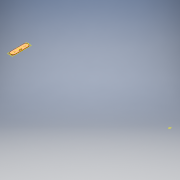
# Autodesk Inventor part: board
Saved by Autodesk Inventor 2017 SP1 (Build 210196100, 196)
## iProperties
Part Number: board
Material: 木材(サクラ)
Document SubType Name: Modeling
Designer: gisen
Density: 0.63 g/cm^3
Appearance: サクラ材 - ナチュラル 抑えた光沢
Mass: 1995.16 g
Surface Area: 3562.51 cm^2
Volume: 3166.92 cm^3
Author: gisen
Autodesk Inventor part; units mm, degrees
ref_plane "作業平面1" through (6614.749, 337.2794, 0) normal (0, 0, 1) x (1, 0, 0)
sketch "スケッチ1" plane through (6614.749, 337.2794, 0) normal (0, 0, 1) x (1, 0, 0)
  line L0 (-6509.749, -42.2794) -> (-6509.749, -632.2794)
  line L1 (-6509.749, -632.2794) -> (-6719.749, -632.2794)
  line L2 (-6719.749, -632.2794) -> (-6719.749, -42.2794)
  line L3 (-6719.749, -42.2794) -> (-6509.749, -42.2794)
  arc A0 (-6509.749, -42.2794) -> (-6719.749, -42.2794) centre (-6614.749, -42.2794) ccw
  arc A1 (-6719.749, -632.2794) -> (-6509.749, -632.2794) centre (-6614.749, -632.2794) ccw
  line L4 (-6614.749, -897.2794) -> (-6614.749, 222.7206) projected
  line L5 (-8036.2537, -337.2794) -> (1179.2797, -337.2794) projected
  line L6 (-6509.749, -337.2794) -> (-137.2251, -337.2794)
  point P0 (-6614.749, -337.2794)
  dimension "d1" = 210
  dimension "d3" = 105
  dimension "d4" = 590
  dimension "d5" = 105
  dimension "d8" = 295
  constraints: 10 end point, 4 point on circle, 2 centre point, 2 parallel, 2 perpendicular, 2 tangent, 1 collinear, 1 midpoint, 1 vertical
  measures "d1" distance of L0.end L1.end
  measures "d3" radius of A0
  measures "d4" distance between parallel lines of L1 L3
  measures "d5" distance between parallel lines of L0 L4
  measures "d8" distance between parallel lines of L6 L1
extrude "押し出し1" add sketch "スケッチ1" along normal blind 20
sketch "スケッチ2" plane through (6614.749, 337.2794, 0) normal (0, 0, -1) x (-1, 0, 0)
  spline S0 degree 3 poles (6630.8363, -557.2765) (6630.8356, -556.4314) (6630.8307, -555.5861) (6630.7821, -551.1548) (6630.6652, -547.5706) (6630.2129, -540.6292) (6629.8924, -537.269) (6629.059, -531.5504) (6628.6277, -529.1809) (6627.5, -524.5004) (6626.8057, -522.1844) (6625.8839, -519.9595) knots -3.785676 -3.785676 -3.785676 -3.785676 -3.532131 -3.532131 -2.4562 -2.4562 -1.444966 -1.444966 -0.722485 -0.722485 0 0 0 0
  spline S1 degree 3 poles (6630.0302, -579.9499) (6630.1435, -578.1819) (6630.247, -576.4134) (6630.4408, -572.7081) (6630.5289, -570.7713) (6630.6019, -568.834) (6630.6759, -566.8669) (6630.7344, -564.8993) (6630.8129, -561.0466) (6630.8346, -559.1616) (6630.8363, -557.2765) knots -2.294162 -2.294162 -2.294162 -2.294162 -1.762693 -1.762693 -1.181069 -1.181069 -1.181069 -0.590534 -0.590534 -0.025021 -0.025021 -0.025021 -0.025021
  spline S2 degree 3 poles (6629.9005, -581.946) (6629.933, -581.4474) (6629.9654, -580.9489) (6629.9979, -580.4504) (6630.0033, -580.367) (6630.0087, -580.2836) (6630.0195, -580.1167) (6630.0249, -580.0333) (6630.0302, -579.9499) knots 0 0 0 0 0.749256 0.749256 0.749256 0.874628 0.874628 1 1 1 1
  ellipse E0 centre (6627.749, -583.7463) end of major axis (6627.749, -580.2108) minor radius 2.5 (6630.249, -583.7463) -> (6629.9005, -581.946) ccw
  line L0 (6630.249, -596.9595) -> (6630.249, -583.7463)
  line L1 (6640.249, -596.9595) -> (6630.249, -596.9595)
  arc A0 (6640.249, -596.9595) -> (6641.749, -595.4595) centre (6640.249, -595.4595) ccw
  line L2 (6641.749, -521.4595) -> (6641.749, -595.4595)
  arc A1 (6641.749, -521.4595) -> (6640.249, -519.9595) centre (6640.249, -521.4595) ccw
  line L3 (6625.8839, -519.9595) -> (6640.249, -519.9595)
  circle A2 centre (6635.249, -591.4595) radius 3
  circle A3 centre (6635.249, -528.4595) radius 3
  circle A4 centre (6594.249, -591.4595) radius 3
  circle A5 centre (6594.249, -528.4595) radius 3
  spline S3 degree 3 poles (6599.4677, -579.9499) (6599.473, -580.0333) (6599.4784, -580.1167) (6599.4892, -580.2836) (6599.4946, -580.367) (6599.5, -580.4504) (6599.5325, -580.9489) (6599.5649, -581.4474) (6599.5974, -581.946) knots 0 0 0 0 0.125372 0.125372 0.250745 0.250745 0.250745 1 1 1 1
  spline S4 degree 3 poles (6598.6616, -557.2765) (6598.6633, -559.1539) (6598.6848, -561.0313) (6598.7628, -564.8687) (6598.8208, -566.8287) (6598.8943, -568.7881) (6598.9673, -570.7332) (6599.0556, -572.6776) (6599.25, -576.3981) (6599.3539, -578.1743) (6599.4677, -579.9499) knots -2.319296 -2.319296 -2.319296 -2.319296 -1.756075 -1.756075 -1.167834 -1.167834 -1.167834 -0.583917 -0.583917 -0.050156 -0.050156 -0.050156 -0.050156
  spline S5 degree 3 poles (6603.614, -519.9595) (6602.3019, -523.1265) (6601.4408, -526.4662) (6600.1974, -532.85) (6599.7845, -535.9073) (6599.0649, -543.0901) (6598.8445, -547.2235) (6598.6873, -553.3316) (6598.6634, -555.3041) (6598.6616, -557.2765) knots -3.810629 -3.810629 -3.810629 -3.810629 -2.782212 -2.782212 -1.858006 -1.858006 -0.616716 -0.616716 -0.024978 -0.024978 -0.024978 -0.024978
  line L4 (6589.249, -519.9595) -> (6603.614, -519.9595)
  arc A6 (6589.249, -519.9595) -> (6587.749, -521.4595) centre (6589.249, -521.4595) ccw
  line L5 (6587.749, -595.4595) -> (6587.749, -521.4595)
  arc A7 (6587.749, -595.4595) -> (6589.249, -596.9595) centre (6589.249, -595.4595) ccw
  line L6 (6599.249, -596.9595) -> (6589.249, -596.9595)
  line L7 (6599.249, -583.7463) -> (6599.249, -596.9595)
  ellipse E1 centre (6601.749, -583.7463) end of major axis (6601.749, -580.2108) minor radius 2.5 (6599.5974, -581.946) -> (6599.249, -583.7463) ccw
  spline S6 degree 3 poles (6630.8363, -107.2765) (6630.8356, -106.4314) (6630.8307, -105.5861) (6630.7821, -101.1548) (6630.6652, -97.5706) (6630.2129, -90.6292) (6629.8924, -87.269) (6629.059, -81.5504) (6628.6277, -79.1809) (6627.5, -74.5004) (6626.8057, -72.1844) (6625.8839, -69.9595) knots -3.785676 -3.785676 -3.785676 -3.785676 -3.532131 -3.532131 -2.4562 -2.4562 -1.444966 -1.444966 -0.722485 -0.722485 0 0 0 0
  spline S7 degree 3 poles (6630.0302, -129.9499) (6630.1435, -128.1819) (6630.247, -126.4134) (6630.4408, -122.7081) (6630.5289, -120.7713) (6630.6019, -118.834) (6630.6759, -116.8669) (6630.7344, -114.8993) (6630.8129, -111.0466) (6630.8346, -109.1616) (6630.8363, -107.2765) knots -2.294162 -2.294162 -2.294162 -2.294162 -1.762693 -1.762693 -1.181069 -1.181069 -1.181069 -0.590534 -0.590534 -0.025021 -0.025021 -0.025021 -0.025021
  spline S8 degree 3 poles (6629.9005, -131.946) (6629.933, -131.4474) (6629.9654, -130.9489) (6629.9979, -130.4504) (6630.0033, -130.367) (6630.0087, -130.2836) (6630.0195, -130.1167) (6630.0249, -130.0333) (6630.0302, -129.9499) knots 0 0 0 0 0.749256 0.749256 0.749256 0.874628 0.874628 1 1 1 1
  ellipse E2 centre (6627.749, -133.7463) end of major axis (6627.749, -130.2108) minor radius 2.5 (6630.249, -133.7463) -> (6629.9005, -131.946) ccw
  line L8 (6630.249, -146.9595) -> (6630.249, -133.7463)
  line L9 (6640.249, -146.9595) -> (6630.249, -146.9595)
  arc A8 (6640.249, -146.9595) -> (6641.749, -145.4595) centre (6640.249, -145.4595) ccw
  line L10 (6641.749, -71.4595) -> (6641.749, -145.4595)
  arc A9 (6641.749, -71.4595) -> (6640.249, -69.9595) centre (6640.249, -71.4595) ccw
  line L11 (6625.8839, -69.9595) -> (6640.249, -69.9595)
  circle A10 centre (6635.249, -141.4595) radius 3
  circle A11 centre (6635.249, -78.4595) radius 3
  circle A12 centre (6594.249, -141.4595) radius 3
  circle A13 centre (6594.249, -78.4595) radius 3
  spline S9 degree 3 poles (6599.4677, -129.9499) (6599.473, -130.0333) (6599.4784, -130.1167) (6599.4892, -130.2836) (6599.4946, -130.367) (6599.5, -130.4504) (6599.5325, -130.9489) (6599.5649, -131.4474) (6599.5974, -131.946) knots 0 0 0 0 0.125372 0.125372 0.250745 0.250745 0.250745 1 1 1 1
  spline S10 degree 3 poles (6598.6616, -107.2765) (6598.6633, -109.1539) (6598.6848, -111.0313) (6598.7628, -114.8687) (6598.8208, -116.8287) (6598.8943, -118.7881) (6598.9673, -120.7332) (6599.0556, -122.6776) (6599.25, -126.3981) (6599.3539, -128.1743) (6599.4677, -129.9499) knots -2.319296 -2.319296 -2.319296 -2.319296 -1.756075 -1.756075 -1.167834 -1.167834 -1.167834 -0.583917 -0.583917 -0.050156 -0.050156 -0.050156 -0.050156
  spline S11 degree 3 poles (6603.614, -69.9595) (6602.3019, -73.1265) (6601.4408, -76.4662) (6600.1974, -82.85) (6599.7845, -85.9073) (6599.0649, -93.0901) (6598.8445, -97.2235) (6598.6873, -103.3316) (6598.6634, -105.3041) (6598.6616, -107.2765) knots -3.810629 -3.810629 -3.810629 -3.810629 -2.782212 -2.782212 -1.858006 -1.858006 -0.616716 -0.616716 -0.024978 -0.024978 -0.024978 -0.024978
  line L12 (6589.249, -69.9595) -> (6603.614, -69.9595)
  arc A14 (6589.249, -69.9595) -> (6587.749, -71.4595) centre (6589.249, -71.4595) ccw
  line L13 (6587.749, -145.4595) -> (6587.749, -71.4595)
  arc A15 (6587.749, -145.4595) -> (6589.249, -146.9595) centre (6589.249, -145.4595) ccw
  line L14 (6599.249, -146.9595) -> (6589.249, -146.9595)
  line L15 (6599.249, -133.7463) -> (6599.249, -146.9595)
  ellipse E3 centre (6601.749, -133.7463) end of major axis (6601.749, -130.2108) minor radius 2.5 (6599.5974, -131.946) -> (6599.249, -133.7463) ccw
  point P0 (6614.749, -337.2794)
  constraints: 4 other
hole "穴1" at (-20.5, -191.1802, 0) at (20.5, -191.1802, 0) at (20.5, -254.1802, 0) at (-20.5, -254.1802, 0) at (-20.5, 258.8198, 0) at (20.5, 258.8198, 0) at (-20.5, 195.8198, 0) at (20.5, 195.8198, 0) direction (0, 0, 1) diameter 5.5 end through all
sketch "スケッチ4" plane through (0, 0, 0) normal (0, 0, 1) x (1, 0, 0)
  circle A0 centre (-20.5, 195.8198) radius 2.75 projected
  circle A1 centre (-20.5, 258.8198) radius 2.75 projected
  circle A2 centre (20.5, -254.1802) radius 2.75 projected
  circle A3 centre (-20.5, -191.1802) radius 2.75 projected
  circle A4 centre (20.5, -191.1802) radius 2.75 projected
  circle A5 centre (-20.5, -254.1802) radius 2.75 projected
  circle A6 centre (20.5, 258.8198) radius 2.75 projected
  circle A7 centre (20.5, 195.8198) radius 2.75 projected
  arc A8 (105, 295) -> (-105, 295) centre (0, 295) ccw projected
  line L0 (-105, 295) -> (-105, -295) projected
  arc A9 (-105, -295) -> (105, -295) centre (0, -295) ccw projected
  line L1 (105, -295) -> (105, 295) projected
  line L2 (65, -50) -> (65, 50)
  line L3 (30, 50) -> (30, -50)
  line L4 (30, -50) -> (65, 50) construction
  line L5 (65, -50) -> (30, 50) construction
  arc A10 (30, -50) -> (65, -50) centre (47.5, -40.3175) ccw
  line L6 (-147, 0) -> (147, 0) projected
  arc A11 (65, 50) -> (30, 50) centre (47.5, 40.3175) ccw
  point P0 (0, 0)
  point P1 (47.5, 0)
  dimension "d16" = 35
  dimension "d17" = 100
  dimension "d18" = 40
  dimension "d19" = 20
  dimension "d20" = 20
  constraints: 8 end point, 4 point on circle, 2 centre point, 2 midpoint, 1 parallel
  measures "d16" distance of L3.start L2.end
  measures "d17" distance of L2.end L2.start
  measures "d18" distance between parallel lines of L1 L2
  measures "d19" radius of A10
  measures "d20" radius of A11
extrude "押し出し2" cut sketch "スケッチ4" along normal through all contours L6 L3 A11 L2 | L2 A10 L3 L6
equation "\"d5\" = 0.5 * d1"
equation "\"d8\" = 0.5 * d4"
equation "\"d20\" = d19"
